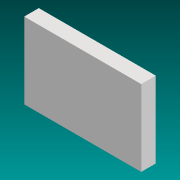
# Autodesk Inventor part: 连接件
Saved by Autodesk Inventor 2021 (Build 250183000, 183)
## iProperties
Created: 2025-04-18
Part Number: 连接件
Material: 常规
Document SubType Name: Modeling
Designer: 86155
Density: 1 g/cm^3
Appearance: 默认
Author: 86155
Autodesk Inventor part; units mm, degrees
ref_plane "YZ Plane" through (0, 0, 0) normal (1, 0, 0) x (0, 1, 0)
ref_plane "XZ Plane" through (0, 0, 0) normal (0, 1, 0) x (-1, 0, 0)
ref_plane "XY Plane" through (0, 0, 0) normal (0, 0, 1) x (1, 0, 0)
sketch "草图1" plane through (0, 0, 0) normal (0, 0, 1) x (1, 0, 0)
  line L0 (0, 0) -> (40, 0)
  line L1 (40, 0) -> (40, -26)
  line L2 (40, -26) -> (0, -26)
  line L3 (0, -26) -> (0, 0)
  dimension "d0" = 40
  dimension "d1" = 26
  constraints: 8 end point, 2 parallel, 1 horizontal, 1 perpendicular
  measures "d0" distance of L1.end L2.end
  measures "d1" distance of L0.end L1.end
extrude "拉伸1" add sketch "草图1" along normal blind 10
ref_plane "工作平面1" through (20, -26, 0) normal (1, 0, 0) x (0, 0, -1)
sketch "草图2" plane through (20, -26, 0) normal (1, 0, 0) x (0, 0, -1)
  line L0 (0, 26) -> (-10, 26) projected
  line L1 (0, 26) -> (-10, 26)
  line L2 (-10, 26) -> (-10, 38)
  line L3 (-10, 38) -> (0, 38)
  line L4 (0, 38) -> (0, 26)
  line L5 (-10, 38) -> (-41, 38)
  line L6 (-41, 38) -> (-41, 34.5)
  line L7 (-41, 34.5) -> (-10, 34.5)
  line L8 (-10, 34.5) -> (-10, 38)
  line L9 (-41, 34.5) -> (-31, 34.5)
  line L10 (-31, 34.5) -> (-31, 30.5)
  line L11 (-31, 30.5) -> (-41, 30.5)
  line L12 (-41, 30.5) -> (-41, 34.5)
  dimension "d5" = 10
  dimension "d6" = 12
  dimension "d7" = 31
  dimension "d8" = 3.5
  dimension "d9" = 10
  dimension "d10" = 4
  constraints: 24 end point, 6 parallel, 3 horizontal, 3 perpendicular
  measures "d5" distance of L2.end L3.end
  measures "d6" distance of L1.end L2.end
  measures "d7" distance of L7.end L6.end
  measures "d8" distance of L6.end L5.end
  measures "d9" distance of L10.end L11.end
  measures "d10" distance of L9.end L10.end
extrude "拉伸2" add sketch "草图2" along normal mid plane 20
sketch "草图3" plane through (0, 0, 0) normal (0, 0, -1) x (-1, 0, 0)
  line L0 (-30, -11) -> (-10, -11)
  line L1 (-10, -11) -> (-10, -15)
  line L2 (-10, -15) -> (-30, -15)
  line L3 (-30, -15) -> (-30, -11)
  line L4 (-40, 0) -> (-30, 0) projected
  line L5 (-40, -26) -> (-40, 0) projected
  line L6 (-30, -11) -> (-10, -11)
  line L7 (-10, -11) -> (-10, -6)
  line L8 (-10, -6) -> (-30, -6)
  line L9 (-30, -6) -> (-30, -11)
  line L10 (-30, -15) -> (-10, -15)
  line L11 (-10, -15) -> (-10, -20)
  line L12 (-10, -20) -> (-30, -20)
  line L13 (-30, -20) -> (-30, -15)
  point P0 (0, 0)
  dimension "d13" = 20
  dimension "d14" = 4
  dimension "d15" = 11
  dimension "d16" = 10
  dimension "d17" = 5
  dimension "d18" = 20
  dimension "d19" = 5
  constraints: 24 end point, 6 parallel, 3 horizontal, 3 perpendicular
  measures "d13" distance of L1.end L2.end
  measures "d14" distance of L0.end L1.end
  measures "d15" distance between parallel lines of L4 L0
  measures "d16" distance between parallel lines of L5 L3
  measures "d17" distance of L7.end L6.end
  measures "d18" distance of L11.end L12.end
  measures "d19" distance between parallel lines of L12 L2
extrude "拉伸3" add sketch "草图3" along normal blind 13 contours L9 L8 L7 L0 | L2 L11 L12 L13
fillet "圆角1" radius 5 6 edges at (30, -8.5, 0) (20, -6, 0) (10, -8.5, 0) (10, -17.5, 0) (20, -20, 0) (30, -17.5, 0)
fillet "圆角2" radius 5 2 edges at (20, 12, 0) (20, 8.5, 10)
